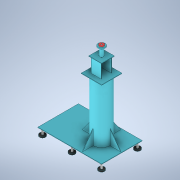
# Autodesk Inventor part: base plate
Saved by Autodesk Inventor 2020 (Build 240168000, 168)
## iProperties
Created: 2020-07-25
Part Number: base plate
Material: Steel, Mild
Document SubType Name: Modeling
Designer: Vikki
Density: 7.85 g/cm^3
Appearance: Cadet Blue
Mass: 6463.25 g
Surface Area: 1561.97 cm^2
Volume: 823.344 cm^3
Author: Vikki
Autodesk Inventor part; units mm, degrees
ref_plane "Work Plane1" through (0, 0, 0) normal (0, 0, 1) x (1, 0, 0)
sketch "Sketch1" plane through (0, 0, 0) normal (0, 0, 1) x (1, 0, 0)
  circle A0 centre (0, 0) radius 9
  line L0 (250, 250) -> (-250, 250)
  line L1 (-250, 250) -> (-250, -250)
  line L2 (-250, -250) -> (250, -250)
  line L3 (250, -250) -> (250, 250)
  line L4 (250, 250) -> (-250, -250) construction
  line L5 (-250, 250) -> (250, -250) construction
  dimension "d0" = 18
  dimension "d1" = 500
  dimension "d2" = 500
  constraints: 12 end point, 2 midpoint, 2 parallel, 1 centre point, 1 coincident, 1 horizontal, 1 perpendicular
  measures "d0" diameter of A0
  measures "d1" distance of L0.start L0.end
  measures "d2" distance of L0.end L1.end
extrude "Extrusion1" add sketch "Sketch1" along normal blind 8
sketch "Sketch3" plane through (0, 0, 0) normal (0, 0, -1) x (-1, 0, 0)
  circle A0 centre (0, 0) radius 9 projected
  circle A1 centre (0, 0) radius 40
  dimension "d5" = 80
  constraints: 1 centre point, 1 coincident
  measures "d5" diameter of A1
extrude "Extrusion2" cut sketch "Sketch3" against normal blind 2.5
ref_plane "Work Plane2" through (-250, 0, 0) normal (0, 1, 0) x (1, 0, 0)
sketch "Sketch6" plane through (0, 0, 8) normal (0, 0, 1) x (1, 0, 0)
  line L0 (-250, -250) -> (250, -250) projected
  line L1 (250, 250) -> (-250, 250) projected
  line L2 (250, -250) -> (250, 250)
  line L3 (250, 250) -> (150, 250)
  line L4 (150, 250) -> (150, -250)
  line L5 (150, -250) -> (250, -250)
  point P0 (0, 0)
  dimension "d22" = 100
  constraints: 8 end point, 2 parallel, 1 perpendicular, 1 vertical
  measures "d22" distance of L3.end L1.start
extrude "Extrusion5" cut sketch "Sketch6" against normal up to surface (8 mm away)
sketch "Sketch7" plane through (0, 0, 8) normal (0, 0, 1) x (1, 0, 0)
  line L0 (-100, -100) -> (100, -100) construction
  line L1 (100, -100) -> (100, 100) construction
  line L2 (100, 100) -> (-100, 100) construction
  line L3 (-100, 100) -> (-100, -100) construction
  line L4 (-100, -100) -> (100, 100) construction
  line L5 (100, -100) -> (-100, 100) construction
  circle A0 centre (100, 100) radius 3
  circle A1 centre (-100, 100) radius 3
  circle A2 centre (-100, -100) radius 3
  circle A3 centre (100, -100) radius 3
  point P0 (0, 0)
  point P1 (0, 0)
  point P2 (0, 0)
  point P3 (0, 0)
  dimension "d25" = 200
  dimension "d26" = 6
  dimension "d29" = 360
  constraints: 12 end point, 4 centre point, 3 coincident, 2 midpoint, 2 parallel, 2 perpendicular, 1 horizontal, 11 other
  measures "d25" distance of L1.end L2.end
  measures "d26" diameter of A0
extrude "Extrusion6" cut sketch "Sketch7" against normal up to surface (8 mm away)
sketch "Sketch8" plane through (0, 0, 2.5) normal (0, 0, -1) x (-1, 0, 0)
  circle A0 centre (0, 0) radius 9 projected
  circle A1 centre (0, 0) radius 40 projected
extrude "Extrusion7" add sketch "Sketch8" along normal blind 17 and the other way blind 2
sketch "Sketch9" plane through (0, 0, 8) normal (0, 0, 1) x (1, 0, 0)
  circle A0 centre (0, 0) radius 9 projected
  circle A1 centre (0, 0) radius 9 projected
  circle A2 centre (0, 0) radius 60
  circle A3 centre (0, 0) radius 500
  dimension "d35" = 120
  dimension "d36" = 1000
  constraints: 2 centre point, 2 coincident
  measures "d35" diameter of A2
  measures "d36" diameter of A3
extrude "Extrusion8" cut sketch "Sketch9" against normal up to surface (8 mm away) contours A3
sketch "Sketch10" plane through (0, 0, 8) normal (0, 0, 1) x (1, 0, 0)
  circle A0 centre (0, 0) radius 9 projected
  circle A1 centre (0, 0) radius 30
  circle A2 centre (0, 0) radius 9 projected
  circle A3 centre (0, 0) radius 9.25
  dimension "d41" = 60
  dimension "d42" = 18.5
  constraints: 2 centre point, 2 coincident
  measures "d41" diameter of A1
  measures "d42" diameter of A3
extrude "Extrusion9" add sketch "Sketch10" along normal blind 150 contours A1
sketch "Sketch11" plane through (0, 0, 8) normal (0, 0, 1) x (1, 0, 0)
  circle A0 centre (0, 0) radius 30 projected
  circle A1 centre (0, 0) radius 30 projected
  circle A2 centre (0, 0) radius 60 projected
extrude "Extrusion10" add sketch "Sketch11" along normal blind 7
sketch "Sketch14" plane through (0, 0, 158) normal (0, 0, 1) x (1, 0, 0)
  line L0 (-110, 110) -> (110, 110)
  line L1 (110, 110) -> (110, -110)
  line L2 (110, -110) -> (-110, -110)
  line L3 (-110, -110) -> (-110, 110)
  line L4 (-110, 110) -> (110, -110) construction
  line L5 (110, 110) -> (-110, -110) construction
  circle A0 centre (0, 0) radius 9.25 projected
  dimension "d48" = 220
  constraints: 12 end point, 2 midpoint, 2 parallel, 2 perpendicular, 1 horizontal
  measures "d48" distance of L0.start L0.end
extrude "Extrusion11" add sketch "Sketch14" along normal blind 8
sketch "Sketch15" plane through (0, 0, 166) normal (0, 0, 1) x (1, 0, 0)
  circle A0 centre (-26.5165, -26.5165) radius 3 projected
  circle A1 centre (-26.5165, 26.5165) radius 3 projected
  circle A2 centre (26.5165, 26.5165) radius 3 projected
  circle A3 centre (26.5165, -26.5165) radius 3 projected
  circle A4 centre (0, 0) radius 22 projected
  arc A5 (42.0269, -5.6127) -> (33.6863, -25.7487) centre (42.4985, -17.6034) ccw projected
  arc A6 (25.7487, -33.6863) -> (33.6863, -25.7487) centre (0, 0) ccw projected
  arc A7 (25.7487, -33.6863) -> (5.6127, -42.0269) centre (17.6034, -42.4985) ccw projected
  arc A8 (-5.6127, -42.0269) -> (5.6127, -42.0269) centre (0, 0) ccw projected
  arc A9 (-5.6127, -42.0269) -> (-25.7487, -33.6863) centre (-17.6034, -42.4985) ccw projected
  arc A10 (-33.6863, -25.7487) -> (-25.7487, -33.6863) centre (0, 0) ccw projected
  arc A11 (-33.6863, -25.7487) -> (-42.0269, -5.6127) centre (-42.4985, -17.6034) ccw projected
  arc A12 (-42.0269, 5.6127) -> (-42.0269, -5.6127) centre (0, 0) ccw projected
  arc A13 (-42.0269, 5.6127) -> (-33.6863, 25.7487) centre (-42.4985, 17.6034) ccw projected
  arc A14 (-25.7487, 33.6863) -> (-33.6863, 25.7487) centre (0, 0) ccw projected
  arc A15 (-25.7487, 33.6863) -> (-5.6127, 42.0269) centre (-17.6034, 42.4985) ccw projected
  arc A16 (5.6127, 42.0269) -> (-5.6127, 42.0269) centre (0, 0) ccw projected
  arc A17 (5.6127, 42.0269) -> (25.7487, 33.6863) centre (17.6034, 42.4985) ccw projected
  arc A18 (33.6863, 25.7487) -> (25.7487, 33.6863) centre (0, 0) ccw projected
  arc A19 (33.6863, 25.7487) -> (42.0269, 5.6127) centre (42.4985, 17.6034) ccw projected
  arc A20 (42.0269, -5.6127) -> (42.0269, 5.6127) centre (0, 0) ccw projected
  point P0 (0, 0)
extrude "Extrusion12" cut sketch "Sketch15" against normal up to surface (8 mm away) contours A0 | A1 | A2 | A3
sketch "Sketch16" plane through (0, 0, 166) normal (0, 0, 1) x (1, 0, 0)
  point P0 (0, 0)
sketch "Sketch17" plane through (0, 0, 166) normal (0, 0, 1) x (1, 0, 0)
  point P0 (0, 0)
sketch "Sketch18" plane through (0, 0, 166) normal (0, 0, 1) x (1, 0, 0)
  circle A0 centre (0, 0) radius 30 projected
  circle A1 centre (0, 0) radius 30 projected
  circle A2 centre (20, 0) radius 3
  circle A3 centre (-10, 17.3205) radius 3
  circle A4 centre (-10, -17.3205) radius 3
  dimension "d53" = 20
  dimension "d54" = 6
  dimension "d57" = 360
  constraints: 3 centre point, 1 horizontal alignment, 7 other
  measures "d53" distance of point (0, 0) A2.centre
  measures "d54" diameter of A2
extrude "Extrusion13" cut sketch "Sketch18" against normal blind 20 contours A2 | A3 | A4
ref_plane "Work Plane3" through (0, 0, 2.5) normal (0, 0, -1) x (-1, 0, 0)
sketch "Sketch20" plane through (0, 0, 2.5) normal (0, 0, -1) x (-1, 0, 0)
  circle A0 centre (0, 0) radius 9 projected
  circle A1 centre (-20, 0) radius 3 projected
  circle A2 centre (10, -17.3205) radius 3 projected
  circle A3 centre (10, 17.3205) radius 3 projected
  circle A4 centre (-26.5165, -26.5165) radius 3 projected
  circle A5 centre (26.5165, 26.5165) radius 3 projected
  circle A6 centre (26.5165, -26.5165) radius 3 projected
  circle A7 centre (-26.5165, 26.5165) radius 3 projected
  line L0 (-110, -110) -> (-110, 110) projected
  line L1 (-110, 110) -> (110, 110) projected
  line L2 (110, 110) -> (110, -110) projected
  line L3 (110, -110) -> (-110, -110) projected
  circle A8 centre (0, 0) radius 9.25 projected
extrude "Extrusion15" cut sketch "Sketch20" against normal blind 20 contours A1 | A2 | A3
thread "Thread2" size "M6x1" class "6H" standard "ANSI Metric M Profile" length 20
thread "Thread3" size "M6x1" class "6H" standard "ANSI Metric M Profile" length 20
thread "Thread4" size "M6x1" class "6H" standard "ANSI Metric M Profile" length 20
sketch "Sketch22" plane through (0, 0, 2.5) normal (0, 0, -1) x (-1, 0, 0)
  circle A0 centre (10, -17.3205) radius 3 projected
  circle A1 centre (10, -17.3205) radius 3 projected
  circle A2 centre (-20, 0) radius 3 projected
  circle A3 centre (-20, 0) radius 3 projected
  circle A4 centre (10, 17.3205) radius 3 projected
  circle A5 centre (10, 17.3205) radius 3 projected
  circle A6 centre (10, 17.3205) radius 5
  circle A7 centre (10, -17.3205) radius 5
  circle A8 centre (-20, 0) radius 5
  point P0 (0, 0)
  dimension "d75" = 10
  constraints: 3 centre point, 2 equal radius
  measures "d75" diameter of A7
extrude "Extrusion16" cut sketch "Sketch22" against normal blind 4
sketch "Sketch23" plane through (0, 0, 166) normal (0, 0, 1) x (1, 0, 0)
  circle A0 centre (0, 0) radius 120 construction
  circle A1 centre (84.8528, 84.8528) radius 8
  circle A2 centre (0, 0) radius 30 projected
  line L0 (0, 0) -> (84.8528, 84.8528) construction
  line L1 (-110, -110) -> (110, -110) projected
  circle A3 centre (-84.8528, 84.8528) radius 8
  circle A4 centre (-84.8528, -84.8528) radius 8
  circle A5 centre (84.8528, -84.8528) radius 8
  line L2 (-84.8528, -84.8528) -> (84.8528, -84.8528)
  line L3 (84.8528, -84.8528) -> (84.8528, -92.8528)
  line L4 (84.8528, -92.8528) -> (-84.8528, -92.8528)
  line L5 (-84.8528, -92.8528) -> (-84.8528, -84.8528)
  line L6 (-84.8528, 84.8528) -> (-84.8528, 92.8528)
  line L7 (-84.8528, 92.8528) -> (84.8528, 92.8528)
  line L8 (84.8528, 92.8528) -> (84.8528, 84.8528)
  line L9 (84.8528, 84.8528) -> (-84.8528, 84.8528)
  dimension "d78" = 240
  dimension "d79" = 16
  dimension "d80" = 45
  dimension "d83" = 360
  dimension "d113" = 8
  dimension "d114" = 8
  constraints: 18 end point, 4 centre point, 4 parallel, 2 perpendicular, 1 coincident, 1 vertical, 12 other
  measures "d79" diameter of A1
  measures "d80" angle of L1 L0
  measures "d113" distance of L4.end L2.start
  measures "d114" distance of L7.end L8.end
extrude "Extrusion17" add sketch "Sketch23" along normal blind 250 contours L8 L9 A1 | A1 L9 A3 L7 | A3 L9 L6 | L2 A5 L4 A4 | A4 L5 L2 | L2 L3 A5 picked at (81.1053, 88.6003) picked at (-81.1053, 88.6003) picked at (-81.1053, -88.6003) picked at (81.1053, -88.6003)
sketch "Sketch24" plane through (84.8528, 84.8528, 416) normal (0, 0, 1) x (1, 0, 0)
  circle A0 centre (-169.7056, 0) radius 8 projected
  circle A1 centre (0, 0) radius 8 projected
  circle A2 centre (0, -169.7056) radius 8 projected
  circle A3 centre (-169.7056, -169.7056) radius 8 projected
  line L0 (25.1472, 25.1472) -> (-194.8528, 25.1472) projected
  line L1 (-194.8528, 25.1472) -> (-194.8528, -194.8528) projected
  line L2 (25.1472, -194.8528) -> (25.1472, 25.1472) projected
  line L3 (-194.8528, -194.8528) -> (25.1472, -194.8528) projected
  line L4 (-259.8528, 90.1472) -> (90.1472, 90.1472)
  line L5 (90.1472, 90.1472) -> (90.1472, -259.8528)
  line L6 (90.1472, -259.8528) -> (-259.8528, -259.8528)
  line L7 (-259.8528, -259.8528) -> (-259.8528, 90.1472)
  point P0 (-84.8528, -84.8528)
  dimension "d89" = 350
  constraints: 8 end point, 3 other
  measures "d89" distance of L4.end L5.end
extrude "Extrusion18" add sketch "Sketch24" along normal blind 8 contours A0 | A1 | A2 | A3 | L2 L3 L1 L0 | L4 L5 L6 L7
sketch "Sketch25" plane through (84.8528, 84.8528, 424) normal (0, 0, 1) x (1, 0, 0)
  circle A0 centre (-84.8528, -84.8528) radius 9.25 projected
  circle A1 centre (-84.8528, -84.8528) radius 150
  circle A2 centre (-84.8528, -84.8528) radius 140
  dimension "d90" = 300
  dimension "d91" = 10
  constraints: 2 centre point, 1 coincident
  measures "d90" diameter of A1
  measures "d91" radial gap between concentric circles of A2 A1
extrude "Extrusion19" add sketch "Sketch25" along normal blind 1000 contours A1
sketch "Sketch26" plane through (0, 0, 1424) normal (0, 0, 1) x (1, 0, 0)
  line L0 (-350, -350) -> (350, -350)
  line L1 (350, -350) -> (350, 350)
  line L2 (350, 350) -> (-350, 350)
  line L3 (-350, 350) -> (-350, -350)
  line L4 (-350, -350) -> (350, 350) construction
  line L5 (350, -350) -> (-350, 350) construction
  line L6 (-350, 350) -> (-750, 350)
  line L7 (-750, 350) -> (-750, -350)
  line L8 (-750, -350) -> (-350, -350)
  line L9 (-350, -350) -> (-350, 350)
  point P0 (0, 0)
  dimension "d94" = 700
  dimension "d97" = 400
  constraints: 20 end point, 4 parallel, 3 perpendicular, 2 horizontal, 2 midpoint
  measures "d94" distance of L1.end L2.end
  measures "d97" distance of L2.end L6.end
extrude "Extrusion20" add sketch "Sketch26" along normal blind 8
sketch "Sketch28" plane through (0, 0, 1432) normal (0, 0, 1) x (1, 0, 0)
  point P0 (0, 0)
sketch "Sketch29" plane through (0, 0, 1432) normal (0, 0, 1) x (1, 0, 0)
  line L0 (-750, -350) -> (350, -350) construction
  line L1 (350, -350) -> (350, 350) construction
  line L2 (350, 350) -> (-750, 350) construction
  line L3 (-750, 350) -> (-750, -350) construction
  line L4 (-710, 310) -> (310, 310) construction
  line L5 (310, 310) -> (310, -310) construction
  line L6 (310, -310) -> (-710, -310) construction
  line L7 (-710, -310) -> (-710, 310) construction
  circle A0 centre (310, 310) radius 15
  circle A1 centre (-710, 310) radius 15
  circle A2 centre (-200, 310) radius 15
  circle A3 centre (-200, -310) radius 15
  circle A4 centre (310, -310) radius 15
  circle A5 centre (-710, -310) radius 15
  circle A6 centre (-200, 0) radius 15
  point P0 (0, 0)
  dimension "d98" = 40
  dimension "d99" = 30
  constraints: 8 end point, 7 centre point, 6 equal radius, 4 coincident, 2 midpoint, 1 horizontal alignment, 1 vertical alignment, 3 other
  measures "d98" distance between parallel lines of L1 L5
  measures "d99" diameter of A0
extrude "Extrusion21" add sketch "Sketch29" along normal blind 100 contours A0 | A1 | A2 | A3 | A4 | A5
sketch "Sketch30" plane through (-200, 0, 1532) normal (0, 0, 1) x (1, 0, 0)
  circle A0 centre (-510, 310) radius 15 construction
  circle A1 centre (0, 310) radius 15 construction
  circle A2 centre (0, -310) radius 15 construction
  circle A3 centre (510, -310) radius 15 construction
  circle A4 centre (510, 310) radius 15 construction
  circle A5 centre (-510, -310) radius 15 construction
  circle A6 centre (-510, 310) radius 50
  circle A7 centre (0, 310) radius 50
  circle A8 centre (510, 310) radius 50
  circle A9 centre (510, -310) radius 50
  circle A10 centre (0, -310) radius 50
  circle A11 centre (-510, -310) radius 50
  point P0 (200, 0)
  dimension "d102" = 100
  constraints: 6 centre point, 5 equal radius
  measures "d102" diameter of A11
extrude "Extrusion22" add sketch "Sketch30" along normal blind 20
ref_plane "Work Plane4" through (-750, 0, 1424) normal (0, 1, 0) x (1, 0, 0)
sketch "Sketch31" plane through (-750, 0, 1424) normal (0, 1, 0) x (1, 0, 0)
  line L0 (900, 1000) -> (900, 0) construction
  line L1 (1100, 0) -> (0, 0) construction
  line L2 (1080, 0) -> (900, 250)
  line L3 (900, 250) -> (880, 277.7778)
  line L4 (880, 277.7778) -> (880, 0)
  line L5 (880, 0) -> (1080, 0)
  point P0 (750, 1424)
  dimension "d105" = 180
  dimension "d106" = 250
  dimension "d107" = 20
  constraints: 8 end point, 3 point on line, 2 collinear, 1 perpendicular
  measures "d105" distance of L2.start L0.end
  measures "d106" distance of L0.end L2.end
  measures "d107" horizontal distance of L0.end L3.end
extrude "Extrusion23" add sketch "Sketch31" along normal mid plane 8
pattern_circular "Circular Pattern1" count 4 over 360 about axis through (0, 0, 424) along (0, 0, 1) of "Extrusion23"
body "Solid1"
